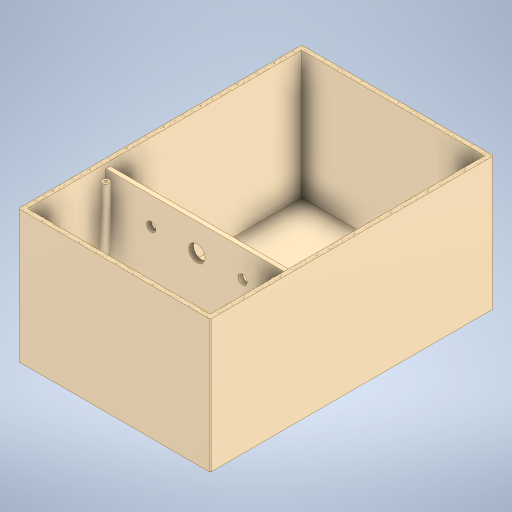
# Autodesk Inventor part: Box
Saved by Autodesk Inventor 2023.1 (Build 271208000, 208)
## iProperties
Created: 2024-03-27
Part Number: Box
Material: Generic
Document SubType Name: Modeling
Designer: bahariridwan
Density: 1 g/cm^3
Appearance: Smooth - Off-White
Author: bahariridwan
Autodesk Inventor part; units mm, degrees
ref_plane "YZ Plane" through (0, 0, 0) normal (1, 0, 0) x (0, 1, 0)
ref_plane "XZ Plane" through (0, 0, 0) normal (0, 1, 0) x (-1, 0, 0)
ref_plane "XY Plane" through (0, 0, 0) normal (0, 0, 1) x (1, 0, 0)
sketch "Sketch4" plane through (0, 0, 0) normal (0, 1, 0) x (-1, 0, 0)
  line L0 (0, 0) -> (210, 0)
  line L1 (210, 0) -> (210, -310)
  line L2 (210, -310) -> (0, -310)
  line L3 (0, -310) -> (0, 0)
  dimension "d9" = 310
  dimension "d10" = 210
  constraints: 8 end point, 2 parallel, 1 horizontal, 1 perpendicular
  measures "d9" distance of L0.end L1.end
  measures "d10" distance of L1.end L2.end
extrude "Extrusion3" add sketch "Sketch4" along normal blind 150
shell "Shell1" thickness 5 removed faces 0
sketch "Sketch5" plane through (-205, 5, -305) normal (1, 0, 0) x (0, 0, -1)
  line L0 (0, 0) -> (-300, 0) projected
  line L1 (-214.5126, 0) -> (-209.5126, 0)
  line L2 (-209.5126, 0) -> (-209.5126, 135)
  line L3 (-209.5126, 135) -> (-214.5126, 135)
  line L4 (-214.5126, 135) -> (-214.5126, 0)
  point P0 (-305, -5)
  point P1 (-209.5126, 0)
  dimension "d18" = 5
  dimension "d19" = 135
  constraints: 8 end point, 2 parallel, 1 horizontal, 1 perpendicular, 1 point on line
  measures "d18" distance of L2.end L3.end
  measures "d19" distance of L1.end L2.end
extrude "Extrusion4" add sketch "Sketch5" along normal blind 200
sketch "Sketch6" plane through (-205, 5, -95.4874) normal (0, 0, -1) x (-1, 0, 0)
  circle A0 centre (-150, 105) radius 5
  circle A1 centre (-100, 105) radius 8.9
  circle A2 centre (-50, 105) radius 5
  line L0 (0, 135) -> (0, 0) projected
  line L1 (0, 135) -> (-200, 135) projected
  point P0 (-205, -5)
  constraints: 3 centre point
chamfer "Chamfer1" distance 1 angle 45 4 edges at (-210, 75, -310) (0, 75, -310) (0, 75, 0) (-210, 75, 0)
extrude "Extrusion5" cut sketch "Sketch6" against normal blind 10
sketch "Sketch7" plane through (-205, 5, -5) normal (0, 1, 0) x (1, 0, 0)
  circle A0 centre (7, 7) radius 4
  circle A1 centre (7, 78.4874) radius 4
  circle A2 centre (193, 7) radius 4
  circle A3 centre (193, 78.4874) radius 4
  line L0 (0, 0) -> (200, 0) projected
  line L1 (200, 0) -> (200, 85.4874) projected
  line L2 (0, 85.4874) -> (200, 85.4874) projected
  line L3 (0, 85.4874) -> (0, 0) projected
  point P0 (205, -5)
  dimension "d37" = 8
  dimension "d38" = 8
  dimension "d39" = 8
  dimension "d40" = 8
  dimension "d41" = 7
  dimension "d42" = 7
  dimension "d43" = 7
  dimension "d44" = 7
  dimension "d45" = 7
  dimension "d46" = 7
  dimension "d47" = 7
  dimension "d48" = 7
  constraints: 4 centre point
  measures "d37" diameter of A1
  measures "d38" diameter of A2
  measures "d39" diameter of A3
  measures "d40" diameter of A0
  measures "d41" distance from line of L0 A2.centre
  measures "d42" distance from line of L1 A2.centre
  measures "d43" distance from line of L1 A3.centre
  measures "d44" distance from line of L2 A3.centre
  measures "d45" distance from line of L0 A0.centre
  measures "d46" distance from line of L3 A0.centre
  measures "d47" distance from line of L3 A1.centre
  measures "d48" distance from line of L2 A1.centre
extrude "Extrusion6" add sketch "Sketch7" along normal blind 130 contours A0 | A1 | A2 | A3
sketch "Sketch8" plane through (-198, 135, -12) normal (0, 1, 0) x (1, 0, 0)
  circle A0 centre (0, 0) radius 1.5
  circle A1 centre (0, 71.4874) radius 4 projected
  circle A2 centre (0, 71.4874) radius 1.5
  circle A3 centre (186, 0) radius 4 projected
  circle A4 centre (186, 0) radius 1.5
  circle A5 centre (186, 71.4874) radius 4 projected
  circle A6 centre (186, 71.4874) radius 1.5
  point P0 (198, -12)
  dimension "d51" = 3
  dimension "d52" = 3
  dimension "d53" = 3
  dimension "d54" = 3
  constraints: 4 centre point, 3 coincident
  measures "d51" diameter of A0
  measures "d52" diameter of A2
  measures "d53" diameter of A4
  measures "d54" diameter of A6
extrude "Extrusion7" cut sketch "Sketch8" against normal blind 30 contours A0 | A2 | A4 | A6
equation "\"d9\" = Panjang_outer"
equation "\"d10\" = Lebar_outer"
equation "\"d11\" = Tinggi_Box"
equation "\"d42\" = d41"
equation "\"d43\" = d41"
equation "\"d44\" = d41"
equation "\"d45\" = d41"
equation "\"d46\" = d41"
equation "\"d47\" = d41"
equation "\"d48\" = d41"
equation "\"Lebar_outer\" = 210"
equation "\"Panjang_outer\" = 310"
equation "\"Tinggi_Box\" = 150"
body "Solid3"
